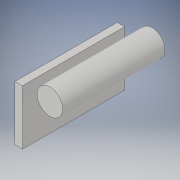
# Autodesk Inventor part: kes
Saved by Autodesk Inventor 2019 (Build 230136000, 136)
## iProperties
Created: 2020-04-03
Part Number: kes
Material: Generic
Document SubType Name: Modeling
Designer: laca
Density: 1 g/cm^3
Appearance: Default
Author: laca
Autodesk Inventor part; units mm, degrees
ref_plane "YZ Plane" through (0, 0, 0) normal (1, 0, 0) x (0, 1, 0)
ref_plane "XZ Plane" through (0, 0, 0) normal (0, 1, 0) x (-1, 0, 0)
ref_plane "XY Plane" through (0, 0, 0) normal (0, 0, 1) x (1, 0, 0)
sketch "Sketch1" plane through (0, 0, 0) normal (0, 0, 1) x (1, 0, 0)
  circle A0 centre (0, 0) radius 25
  line L0 (-25, 0) -> (-25, -117.3669)
  line L1 (0, 0) -> (-53.6656, 0)
  line L2 (-53.6656, 0) -> (-53.6656, -107.3313)
  line L3 (-25, -117.3669) -> (0, 0)
  line L4 (-53.6656, -107.3313) -> (0, 0)
  line L5 (-53.6656, 0) -> (0, 0)
  line L6 (-53.6656, 0) -> (-68.1249, 0)
  line L7 (-68.1249, 0) -> (-68.1249, -107.3313)
  line L8 (-68.1249, -107.3313) -> (-53.6656, -107.3313)
  line L9 (-53.6656, -107.3313) -> (-53.6656, 0)
  dimension "d0" = 50
  dimension "d3" = 120
  dimension "d4" = 120
  constraints: 20 end point, 3 horizontal, 2 parallel, 2 vertical, 1 coincident, 1 horizontal alignment, 1 perpendicular, 2 other
  measures "d3" distance of L0.end L1.start
  measures "d4" distance of L2.end L1.start
extrude "Extrusion1" add sketch "Sketch1" along normal blind 200 contours A0 L3 L1 | L1 L4 A0 | A0 L4 L3 | L2 L8 L7 L6
body "Solid1"
